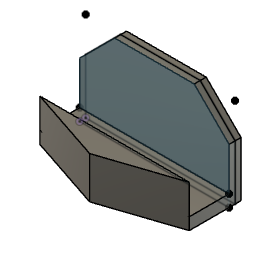
3d16 v1 (Autodesk Fusion 360 design; units mm, degrees)
Autodesk Fusion 360 part; units mm, degrees
sketch "Sketch1" plane through (0, 0, 0) normal (0, 0, 1) x (1, 0, 0)
  line L0 (0, 0) -> (150, 0)
  line L1 (0, 0) -> (0, 55)
  line L2 (35, 90) -> (115, 90)
  line L3 (150, 55) -> (150, 0)
  line L4 (0, 55) -> (35, 90)
  line L5 (150, 55) -> (115, 90)
  point P0 (0, 90)
  point P1 (150, 90)
  dimension "d1" = 150
  dimension "d2" = 90
  dimension "d3" = 35
  dimension "d4" = 35
  dimension "d5" = 35
  dimension "d6" = 35
  constraint coincident L0.start L1.start
  constraint horizontal L0
  constraint vertical L1
  constraint perpendicular L1 L2
  constraint perpendicular L2 L3
  constraint coincident P0 L1
  constraint coincident P0 L2
  constraint coincident P1 L3
  constraint coincident P1 L2
  measures "d1" distance of L0.start L0.end
  measures "d2" distance of L0.start P0
  measures "d3" distance of P0 L1.end
  measures "d4" distance of P0 L2.start
  measures "d5" distance of P1 L3.start
  measures "d6" distance of P1 L2.end
extrude "Extrude1" add sketch "Sketch1" along normal mid plane 12
sketch "Sketch2" plane through (0, 0, 6) normal (0, 0, 1) x (1, 0, 0)
  line L0 (0, 0) -> (150, 0)
  line L1 (150, 0) -> (150, 55)
  line L2 (150, 55) -> (115, 90)
  line L3 (115, 90) -> (35, 90)
  line L4 (35, 90) -> (0, 55)
  line L5 (0, 55) -> (0, 0)
  line L6 (0, 12) -> (150, 12)
  line L7 (150, 0) -> (0, 0)
  dimension "d9" = 12
  constraint coincident L5 L6.start
  constraint coincident L1 L6.end
  constraint perpendicular L1 L6
  constraint coincident L0.end L1.start
  constraint coincident L0.start L5.end
  measures "d9" distance of L6 L7
extrude "Extrude2" add sketch "Sketch2" along normal blind 40 contours L0 L1 L5 L6 L7
sketch "Sketch3" plane through (0, 12, 0) normal (0, 1, 0) x (-1, 0, 0)
  line L0 (-150, 6) -> (0, 6)
  line L1 (0, 6) -> (0, 46)
  line L2 (0, 46) -> (-150, 46)
  line L3 (-150, 46) -> (-150, 6)
  line L4 (0, 46) -> (-75, 71)
  line L5 (-75, 71) -> (-150, 46)
  line L6 (-75, 11.1392) -> (-75, 80.8608)
  dimension "d12" = 25
  dimension "d13" = 25
  constraint coincident L1.end L2.start
  constraint coincident L2.end L3.start
  constraint vertical L6
  constraint midpoint L2 L6
  constraint coincident L4.end L6
  measures "d12" vertical distance of L4.end L2.end
  measures "d13" vertical distance of L1.end L4.end
extrude "Extrude3" add sketch "Sketch3" against normal blind 12 contours L2 L5 L6 | L2 L4 L6
sketch "Sketch4" plane through (0, 0, 6) normal (0, 0, 1) x (1, 0, 0)
  line L0 (0, 12) -> (150, 12)
  line L1 (150, 12) -> (150, 55)
  line L2 (150, 55) -> (115, 90)
  line L3 (115, 90) -> (35, 90)
  line L4 (35, 90) -> (0, 55)
  line L5 (0, 55) -> (0, 12)
sketch "Sketch5" plane through (0, 0, 0) normal (1, 0, 0) x (0, 0, -1)
extrude "Extrude4" add sketch "Sketch3" along normal blind 30 contours L2 L5 L6 | L2 L4 L6
